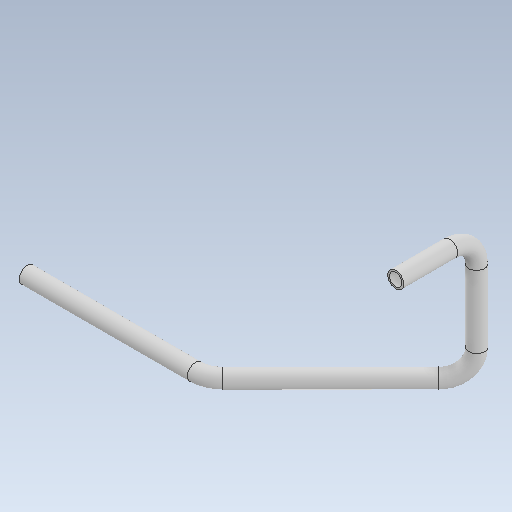
# Autodesk Inventor part: Peça25
Saved by Autodesk Inventor 2021 (Build 250183000, 183)
## iProperties
Category: 41
Created: 2021-07-19
Part Number: Peça25
Material: Genérico
Document SubType Name: Modeling
Designer: Giovanni
Density: 1 g/cm^3
Appearance: Padrão
User Status: 1:6
Author: Giovanni
Keywords: 41
Autodesk Inventor part; units mm, degrees
ref_plane "YZ Plane" through (0, 0, 0) normal (1, 0, 0) x (0, 1, 0)
ref_plane "XZ Plane" through (0, 0, 0) normal (0, 1, 0) x (-1, 0, 0)
ref_plane "XY Plane" through (0, 0, 0) normal (0, 0, 1) x (1, 0, 0)
sketch "Esboço1" plane through (0, 0, 0) normal (0, 0, 1) x (1, 0, 0)
  circle A0 centre (0, 0) radius 7
  circle A1 centre (0, 0) radius 9
  dimension "d0" = 14
  dimension "d1" = 18
  constraints: 2 centre point, 2 coincident
  measures "d0" diameter of A0
  measures "d1" diameter of A1
sketch "Esboço1 outline for Extrusão1" plane through (0, 0, 0) normal (0, 0, 1) x (1, 0, 0)
  circle A0 centre (0, 0) radius 9
  circle A1 centre (0, 0) radius 7
extrude "Extrusão1" add sketch "Esboço1 outline for Extrusão1" against normal blind 60
sketch "Esboço8" plane through (0, 0, -60) normal (0, 0, -1) x (-1, 0, 0)
  circle A0 centre (0, 0) radius 9 projected
  circle A1 centre (0, 0) radius 7 projected
  line L0 (0, 0) -> (0, -30)
  line L1 (-15, -30) -> (15, -30)
  dimension "d18" = 30
  dimension "d19" = 30
  constraints: 4 end point, 1 horizontal, 1 midpoint, 1 vertical
  measures "d18" distance of L0.end L0.start
  measures "d19" distance of L1.start L1.end
sketch "Esboço8 outline for Revolução4" plane through (0, 0, -60) normal (0, 0, -1) x (-1, 0, 0)
  circle A0 centre (0, 0) radius 9
  circle A1 centre (0, 0) radius 7
revolve "Revolução4" add sketch "Esboço8 outline for Revolução4" angle 90 about axis through (15, -30, -60) along (-1, 0, 0)
sketch "Esboço9" plane through (0, -30, -90) normal (0, -1, 0) x (1, 0, 0)
  circle A0 centre (0, 0) radius 9 projected
  circle A1 centre (0, 0) radius 7 projected
  point P0 (0, 90)
sketch "Esboço9 outline for Extrusão3" plane through (0, -30, -90) normal (0, -1, 0) x (1, 0, 0)
  circle A0 centre (0, 0) radius 9
  circle A1 centre (0, 0) radius 7
extrude "Extrusão3" add sketch "Esboço9 outline for Extrusão3" along normal blind 80
sketch "Esboço10" plane through (0, -110, -90) normal (0, -1, 0) x (1, 0, 0)
  circle A0 centre (0, 0) radius 9
  circle A1 centre (0, 0) radius 7
  line L0 (0, 0) -> (-21.213203, 21.213203)
  line L1 (0, 0) -> (0, 30)
  line L2 (-10.606602, 31.819805) -> (-31.819805, 10.606602)
  point P0 (0, 90)
  dimension "d23" = 30
  dimension "d24" = 45
  dimension "d25" = 30
  dimension "d26" = 30
  constraints: 6 end point, 1 midpoint, 1 perpendicular, 1 vertical
  measures "d23" distance of L0.end L0.start
  measures "d24" angle of L1 L0
  measures "d25" distance of L0.start L1.end
  measures "d26" distance of L2.start L2.end
sketch "Esboço10 outline for Revolução5" plane through (0, -110, -90) normal (0, -1, 0) x (1, 0, 0)
  circle A0 centre (0, 0) radius 9
  circle A1 centre (0, 0) radius 7
revolve "Revolução5" add sketch "Esboço10 outline for Revolução5" angle 90 about axis through (-10.606602, -110, -58.180195) along (-0.7071068, 0, -0.7071068)
sketch "Esboço11" plane through (-21.213203, -140, -68.786797) normal (-0.7071068, 0, 0.7071068) x (0.7071068, 0, 0.7071068)
  circle A0 centre (0, 0) radius 9 projected
  circle A1 centre (0, 0) radius 7 projected
  point P0 (63.63961, 140)
sketch "Esboço11 outline for Extrusão4" plane through (-21.213203, -140, -68.786797) normal (-0.7071068, 0, 0.7071068) x (0.7071068, 0, 0.7071068)
  circle A0 centre (0, 0) radius 9
  circle A1 centre (0, 0) radius 7
extrude "Extrusão4" add sketch "Esboço11 outline for Extrusão4" along normal blind 170
sketch "Esboço12" plane through (-141.421356, -140, 51.421356) normal (-0.7071068, 0, 0.7071068) x (0.7071068, 0, 0.7071068)
  circle A0 centre (0, 0) radius 9 projected
  circle A1 centre (0, 0) radius 7 projected
  line L0 (0, 0) -> (-30, 0)
  line L1 (-30, 15) -> (-30, -15)
  point P0 (63.63961, 140)
  dimension "d30" = 30
  dimension "d31" = 30
  constraints: 4 end point, 1 horizontal, 1 midpoint, 1 perpendicular, 1 vertical
  measures "d30" distance of L0.end L0.start
  measures "d31" distance of L1.start L1.end
sketch "Esboço12 outline for Revolução6" plane through (-141.421356, -140, 51.421356) normal (-0.7071068, 0, 0.7071068) x (0.7071068, 0, 0.7071068)
  circle A0 centre (0, 0) radius 9
  circle A1 centre (0, 0) radius 7
revolve "Revolução6" add sketch "Esboço12 outline for Revolução6" angle 45 about axis through (-162.63456, -125, 30.208153) along (0, -1, 0)
sketch "Esboço13" plane through (-162.63456, -140, 60.208153) normal (-1, 0, 0) x (0, 0, 1)
  circle A0 centre (0, 0) radius 9 projected
  circle A1 centre (0, 0) radius 7 projected
  point P0 (-60.208153, 140)
sketch "Esboço13 outline for Extrusão5" plane through (-162.63456, -140, 60.208153) normal (-1, 0, 0) x (0, 0, 1)
  circle A0 centre (0, 0) radius 9
  circle A1 centre (0, 0) radius 7
extrude "Extrusão5" add sketch "Esboço13 outline for Extrusão5" along normal blind 187
